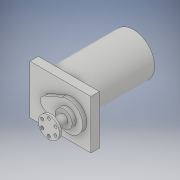
# Autodesk Inventor part: drivemotors
Saved by Autodesk Inventor 2019 (Build 230136000, 136)
## iProperties
Created: 2018-08-20
Part Number: drivemotors
Material: Generic
Document SubType Name: Modeling
Designer: Kitte_X
Density: 1 g/cm^3
Appearance: Default
Author: Kitte_X
Autodesk Inventor part; units mm, degrees
ref_plane "YZ Plane" through (0, 0, 0) normal (1, 0, 0) x (0, 1, 0)
ref_plane "XZ Plane" through (0, 0, 0) normal (0, 1, 0) x (-1, 0, 0)
ref_plane "XY Plane" through (0, 0, 0) normal (0, 0, 1) x (1, 0, 0)
sketch "Sketch1" plane through (0, 0, 0) normal (0, 0, 1) x (1, 0, 0)
  circle A0 centre (0, 0) radius 50
  dimension "d0" = 100
  constraints: 1 centre point, 1 coincident
  measures "d0" diameter of A0
extrude "Extrusion1" add sketch "Sketch1" against normal blind 175
sketch "Sketch2" plane through (0, 0, 0) normal (0, 0, 1) x (1, 0, 0)
  line L0 (94.5, 57.9363) -> (94.5, -57.9363)
  line L1 (94.5, -57.9363) -> (-50, -57.9363)
  line L2 (-50, -57.9363) -> (-50, 57.9363)
  line L3 (-50, 57.9363) -> (94.5, 57.9363)
  circle A0 centre (0, 0) radius 50 projected
  point P0 (94.5, 0)
  dimension "d3" = 144.5
  dimension "d4" = 115.8726
  constraints: 8 end point, 3 perpendicular, 1 horizontal alignment, 1 midpoint, 1 tangent, 1 vertical
  measures "d3" distance between parallel lines of L0 L2
  measures "d4" distance between parallel lines of L1 L3
extrude "Extrusion2" add sketch "Sketch2" along normal blind 20 contours A0 | L0 L1 L2 L3
sketch "Sketch3" plane through (0, 0, 20) normal (0, 0, 1) x (1, 0, 0)
  arc A0 (-6, 13.7477) -> (-6, -13.7477) centre (0, 0) ccw
  arc A1 (36, -32.078) -> (36, 32.078) centre (50, 0) ccw
  line L0 (-6, 13.7477) -> (36, 32.078)
  line L1 (-6, -13.7477) -> (36, -32.078)
  dimension "d8" = 30
  dimension "d9" = 70
  constraints: 5 tangent, 4 end point, 4 point on circle, 2 centre point, 1 coincident
  measures "d8" diameter of A0
  measures "d9" diameter of A1
extrude "Extrusion3" add sketch "Sketch3" along normal blind 10
sketch "Sketch4" plane through (0, 0, 30) normal (0, 0, 1) x (1, 0, 0)
  arc A0 (36, -32.078) -> (36, 32.078) centre (50, 0) ccw projected
  circle A1 centre (50, 0) radius 20
  point P0 (0, 0)
  dimension "d12" = 40
  constraints: 1 centre point, 1 coincident
  measures "d12" diameter of A1
extrude "Extrusion4" add sketch "Sketch4" along normal blind 10
sketch "Sketch5" plane through (50, 0, 40) normal (0, 0, 1) x (1, 0, 0)
  circle A0 centre (-50, 0) radius 50 projected
  circle A1 centre (0, 0) radius 10
  point P0 (-100, 0)
  dimension "d15" = 20
  constraints: 1 centre point, 1 point on circle
  measures "d15" diameter of A1
extrude "Extrusion5" add sketch "Sketch5" along normal blind 30 contours A0 A1 | A0 A1 picked at (-3.2709, -1.921) picked at (2.9235, -2.6438)
sketch "Sketch6" plane through (50, 0, 70) normal (0, 0, 1) x (1, 0, 0)
  circle A0 centre (0, 0) radius 25
  circle A1 centre (0, 18) radius 3.75
  circle A2 centre (-15.5885, 9) radius 3.75
  circle A3 centre (-15.5885, -9) radius 3.75
  circle A4 centre (0, -18) radius 3.75
  circle A5 centre (15.5885, -9) radius 3.75
  circle A6 centre (15.5885, 9) radius 3.75
  point P0 (-50, 0)
  dimension "d18" = 50
  dimension "d19" = 7.5
  dimension "d20" = 18
  dimension "d23" = 360
  constraints: 7 centre point, 1 coincident, 13 other
  measures "d18" diameter of A0
  measures "d19" diameter of A1
  measures "d20" distance of A0.centre A1.centre
extrude "Extrusion6" add sketch "Sketch6" along normal blind 5
body "Solid1"
